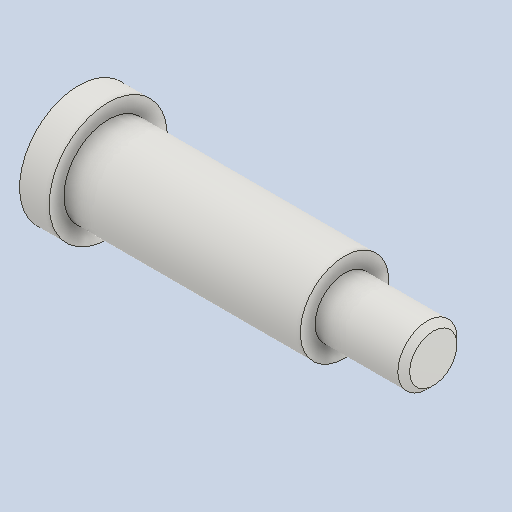
# Autodesk Inventor part: Вал
Saved by Autodesk Inventor 2022 (Build 260153000, 153)
## iProperties
Created: 2021-10-26
Part Number: Вал
Material: Steel
Document SubType Name: Modeling
Designer: RaNSiD
Density: 1 g/cm^3
Appearance: Steel
CustomPartVersion: 1
Author: RaNSiD
Length: 120,000 мм
Autodesk Inventor part; units mm, degrees
ref_plane "Начальная плоскость" through (0, 0, 0) normal (1, 0, 0) x (0, 1, 0)
ref_plane "XZ Plane" through (0, 0, 0) normal (0, 1, 0) x (-1, 0, 0)
ref_plane "XY Plane" through (0, 0, 0) normal (0, 0, 1) x (1, 0, 0)
sketch "Основной эскиз" plane through (0, 0, 0) normal (0, 0, 1) x (1, 0, 0)
  line L0 (0, 0) -> (120, 0)
  line L1 (0, 0) -> (0, 20)
  line L2 (10, 20) -> (10, 15)
  line L3 (0, 20) -> (10, 20)
  line L4 (90, 15) -> (90, 10)
  line L5 (10, 15) -> (90, 15)
  line L6 (120, 10) -> (120, 0)
  line L7 (90, 10) -> (120, 10)
  dimension "d3" = 40
  dimension "d4" = 30
  dimension "d5" = 20
  constraints: 16 end point, 5 horizontal, 4 vertical
  measures "d3" diameter of L3 L0
  measures "d4" diameter of L5 L0
  measures "d5" diameter of L7 L0
revolve "Вращение1" add sketch "Основной эскиз" angle 360 about axis through (0, 0, 0) along (1, 0, 0)
chamfer "Фаска1" distance 2 angle 45 1 edges at (120, -10, 0) measured on face at (119.5, -10, 0)
